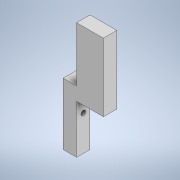
# Autodesk Inventor part: lever staggered
Saved by Autodesk Inventor 2020.2 (Build 242310000, 310)
## iProperties
Created: 2020-02-28
Part Number: lever staggered
Material: Generic
Document SubType Name: Modeling
Designer: ColinP
Density: 1 g/cm^3
Appearance: Default
Author: ColinP
Autodesk Inventor part; units mm, degrees
ref_plane "YZ Plane" through (0, 0, 0) normal (1, 0, 0) x (0, 1, 0)
ref_plane "XZ Plane" through (0, 0, 0) normal (0, 1, 0) x (-1, 0, 0)
ref_plane "XY Plane" through (0, 0, 0) normal (0, 0, 1) x (1, 0, 0)
sketch "Sketch1" plane through (0, 0, 0) normal (0, 0, 1) x (1, 0, 0)
  line L0 (-8.0472, -28.1521) -> (1.9528, -28.1521)
  line L1 (1.9528, -28.1521) -> (1.9528, -64.3521)
  line L2 (1.9528, -64.3521) -> (-8.0472, -64.3521)
  line L3 (-8.0472, -64.3521) -> (-8.0472, -28.1521)
  point P0 (0, 0)
  dimension "d0" = 10
  dimension "d1" = 36.2
  constraints: 8 end point, 2 parallel, 1 horizontal, 1 perpendicular
  measures "d0" distance of L1.end L2.end
  measures "d1" distance of L0.end L1.end
extrude "Extrusion1" add sketch "Sketch1" along normal blind 10
sketch "Sketch3" plane through (1.9528, -64.3521, 0) normal (1, 0, 0) x (0, 0, -1)
  line L0 (0, 36.2) -> (-10, 36.2) projected
  line L1 (-5, 36.2) -> (-5, 26.2)
  point P0 (0, 64.3521)
  dimension "d12" = 10
  constraints: 2 end point, 1 midpoint, 1 vertical
  measures "d12" distance of L1.start L1.end
hole "Hole2" at (1.9528, -38.1521, 5) direction (-1, 0, 0) diameter 3.6 end through all clearance for "Flat Head Machine Screw" size "M3" standard "Ansi Metric M Profile"
sketch "Sketch4" plane through (-8.0472, -28.1521, 0) normal (0, 1, 0) x (1, 0, 0)
  line L0 (10, -10) -> (0, -10) projected
  line L1 (10, 0) -> (10, -10) projected
  line L2 (0, -10) -> (10, -10)
  line L3 (10, -10) -> (10, 0)
  line L4 (10, 0) -> (0, 0)
  line L5 (0, 0) -> (0, -10)
  point P0 (8.0472, 0)
  constraints: 8 end point, 2 parallel, 1 horizontal, 1 perpendicular
extrude "Extrusion2" add sketch "Sketch4" along normal blind 10
sketch "Sketch5" plane through (1.9528, -64.3521, 10) normal (1, 0, 0) x (0, 0, -1)
  line L0 (0, 0) -> (0, 46.2) projected
  line L1 (0, 46.2) -> (10, 46.2)
  line L2 (10, 46.2) -> (10, 36.2)
  line L3 (10, 36.2) -> (0, 36.2)
  line L4 (0, 36.2) -> (0, 46.2)
  point P0 (10, 64.3521)
  dimension "d22" = 10
  dimension "d23" = 10
  constraints: 8 end point, 2 parallel, 1 horizontal, 1 perpendicular
  measures "d22" distance of L2.end L3.end
  measures "d23" distance of L1.end L2.end
extrude "Extrusion3" add sketch "Sketch5" along normal blind 20
sketch "Sketch6" plane through (-8.0472, -18.1521, 0) normal (0, 1, 0) x (1, 0, 0)
  line L0 (0, -10) -> (30, -10) projected
  line L1 (10, 0) -> (30, 0)
  line L2 (30, 0) -> (30, -10)
  line L3 (30, -10) -> (10, -10)
  line L4 (10, -10) -> (10, 0)
  point P0 (8.0472, 0)
  point P1 (10, -10)
  constraints: 8 end point, 2 parallel, 1 horizontal, 1 perpendicular
extrude "Extrusion4" add sketch "Sketch6" along normal blind 50.8
sketch "Sketch7" plane through (-8.0472, 32.6479, 0) normal (0, 1, 0) x (1, 0, 0)
  line L0 (30, 0) -> (10, 0) projected
  line L1 (10, 0) -> (10, -10) projected
  line L2 (10, -10) -> (30, -10) projected
  line L3 (30, -10) -> (30, 0) projected
  point P0 (8.0472, 0)
extrude "Extrusion5" cut sketch "Sketch7" against normal blind 10
body "Solid1"
